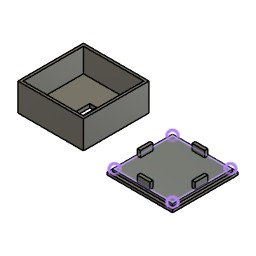
caja control servo_ (Autodesk Fusion 360 design; units mm, degrees)
Autodesk Fusion 360 part; units mm, degrees
sketch "Sketch1" plane through (0, 0, 0) normal (0, 1, 0) x (1, 0, 0)
  line L0 (-58.5421, 52.4156) -> (41.4579, 52.4156)
  line L1 (41.4579, 52.4156) -> (41.4579, -47.5844)
  line L2 (41.4579, -47.5844) -> (-58.5421, -47.5844)
  line L3 (-58.5421, -47.5844) -> (-58.5421, 52.4156)
  dimension "d1" = 100
  dimension "d2" = 100
  constraint horizontal L0
  constraint vertical L1
  constraint horizontal L2
  constraint vertical L3
  measures "d1" distance of L0.start L0.end
  measures "d2" distance of L0.start L2.end
extrude "Extrude1" add sketch "Sketch1" along normal blind 40 makes body 1
shell "Shell1" thickness 2 outward thickness 2 removed faces 1 at (-25.2087, 40, -19.0822) on bodies 1
sketch "Sketch2" plane through (0, 2, 0) normal (0, 1, 0) x (-1, 0, 0)
  line L0 (56.5421, 45.5844) -> (-39.4579, 45.5844)
  line L1 (-39.4579, 45.5844) -> (-39.4579, -50.4156)
  line L2 (-39.4579, -50.4156) -> (56.5421, -50.4156)
  line L3 (56.5421, -50.4156) -> (56.5421, 45.5844)
  line L4 (0.5421, 9.5844) -> (0.5421, -14.4156)
  line L5 (8.5421, 9.5844) -> (0.5421, 9.5844)
  line L6 (8.5421, -14.4156) -> (0.5421, -14.4156)
  line L7 (8.5421, 9.5844) -> (8.5421, -14.4156)
extrude "Extrude2" cut sketch "Sketch2" against normal blind 20 contours L4 L5 L6 L7 bodies 1
extrude "Extrude3" add 1 faces at (-43.2087, -2, -6.4156) along direction (0, -1, 0) blind 2 on bodies 1 bodies 1
sketch "Sketch4" plane through (0, 0, 0) normal (0, 1, 0) x (1, 0, 0)
  line L0 (80, 50) -> (180, 50)
  line L1 (180, 50) -> (180, -50)
  line L2 (180, -50) -> (80, -50)
  line L3 (80, -50) -> (80, 50)
  dimension "d13" = 100
  dimension "d14" = 100
  constraint horizontal L0
  constraint vertical L1
  constraint horizontal L2
  constraint vertical L3
  measures "d13" distance of L0.start L0.end
  measures "d14" distance of L0.start L2.end
extrude "Extrude4" add sketch "Sketch4" along normal blind 2 separate body makes body 2
sketch "Sketch5" plane through (0, 2, 0) normal (0, 1, 0) x (-1, 0, 0)
  line L0 (-80, 50) -> (-180, 50)
  line L1 (-180, 50) -> (-180, -50)
  line L2 (-180, -50) -> (-80, -50)
  line L3 (-80, -50) -> (-80, 50)
  line L4 (-84, 46) -> (-176, 46)
  line L5 (-176, 46) -> (-176, -46)
  line L6 (-176, -46) -> (-84, -46)
  line L7 (-84, -46) -> (-84, 46)
  dimension "d17" = -4
extrude "Extrude5" add sketch "Sketch5" along normal blind 4 contours L4 L5 L6 L7 bodies 2
extrude "Extrude6" add 1 faces at (113.3333, 0, -16.6667) along direction (0, -1, 0) blind 2 on bodies 2 bodies 2
copy_body "Body->Comp1" bodies 2 removing the originals makes body 3 in component "Component"
copy_body "Body->Comp2" bodies 1 removing the originals makes body 4 in component "Component'"
sketch "Sketch6" plane through (0, 6, 0) normal (0, 1, 0) x (-1, 0, 0)
  line L0 (-84, -46) -> (-84, 46)
  line L1 (-84, 46) -> (-176, 46)
  line L2 (-176, 46) -> (-176, -46)
  line L3 (-176, -46) -> (-84, -46)
sketch "Sketch7" plane through (0, 6, 0) normal (0, 1, 0) x (-1, 0, 0)
  line L0 (-84, -46) -> (-84, 46)
  line L1 (-84, 0) -> (-84, -10)
  line L2 (-84, -10) -> (-89, -10)
  line L3 (-89, -10) -> (-89, 10)
  line L4 (-89, 10) -> (-84, 10)
  line L5 (-84, 10) -> (-84, -10)
  dimension "d22" = 10
  dimension "d23" = 5
  dimension "d24" = 20
  constraint midpoint L0 L1.start
  constraint parallel L0 L1
  constraint horizontal L2
  constraint vertical L3
  constraint horizontal L4
  constraint vertical L5
  measures "d22" distance of L1.start L1.end
  measures "d23" distance of L1.end L2.end
  measures "d24" distance of L1.end L4.end
extrude "Extrude7" add sketch "Sketch7" along normal blind 10 separate body makes body 5
sketch "Sketch8" plane through (0, 6, 0) normal (0, 1, 0) x (-1, 0, 0)
  line L0 (-176, -46) -> (-84, -46)
  line L1 (-84, 46) -> (-176, 46)
sketch "Sketch9" plane through (0, 6, 0) normal (0, 1, 0) x (-1, 0, 0)
  line L0 (-84, -46) -> (-84, 46)
  line L1 (-176, 46) -> (-176, -46)
sketch "Sketch10" plane through (0, 6, 0) normal (0, 1, 0) x (-1, 0, 0)
  line L0 (-130, -46) -> (-120, -46)
  line L1 (-120, -46) -> (-140, -46)
  line L2 (-140, -46) -> (-140, -41)
  line L3 (-140, -41) -> (-120, -41)
  line L4 (-120, -41) -> (-120, -46)
  line L5 (-176, 0) -> (-176, -10)
  line L6 (-176, -10) -> (-171, -10)
  line L7 (-171, -10) -> (-171, 10)
  line L8 (-171, 10) -> (-176, 10)
  line L9 (-176, 10) -> (-176, -10)
  line L10 (-130, 46) -> (-140, 46)
  line L11 (-140, 46) -> (-120, 46)
  line L12 (-120, 46) -> (-120, 41)
  line L13 (-120, 41) -> (-140, 41)
  line L14 (-140, 41) -> (-140, 46)
  point P0 (-130, -46)
  point P1 (-176, 0)
  point P2 (-130, 46)
  dimension "d27" = 10
  dimension "d28" = 20
  dimension "d29" = 5
  dimension "d30" = 10
  dimension "d31" = 5
  dimension "d32" = 20
  dimension "d33" = 10
  dimension "d34" = 20
  dimension "d35" = 5
  constraint coincident P0 L0.start
  constraint horizontal L1
  constraint vertical L2
  constraint horizontal L3
  constraint vertical L4
  constraint coincident P1 L5.start
  constraint perpendicular L1 L5
  constraint horizontal L6
  constraint vertical L7
  constraint horizontal L8
  constraint vertical L9
  constraint coincident P2 L10.start
  constraint horizontal L11
  constraint vertical L12
  constraint horizontal L13
  constraint vertical L14
  measures "d27" distance of P0 L0.end
  measures "d28" distance of L0.end L1.end
  measures "d29" distance of L0.end L3.end
  measures "d30" distance of P1 L5.end
  measures "d31" distance of L5.end L6.end
  measures "d32" distance of L5.end L8.end
  measures "d33" distance of P2 L10.end
  measures "d34" distance of L10.end L11.end
  measures "d35" distance of L10.end L13.end
extrude "Extrude8" add sketch "Sketch10" along normal blind 10 separate body makes body 6 at (126.6667, 9.3333, -46) makes body 7 at (176, 9.3333, 3.3333) makes body 8 at (133.3333, 9.3333, 46)
extrude "Extrude1'" add 1 faces at (80, 0.6667, 16.6667) along direction (-1, 0, 0) blind 2 on bodies 3 bodies 3 in component "Component"
extrude "Extrude2'" add 1 faces at (180, -0.6667, 16.6667) along direction (1, 0, 0) blind 2 on bodies 3 bodies 3 in component "Component"
extrude "Extrude3'" add 1 faces at (112.6667, 0.6667, 50) along direction (0, 0, 1) blind 2 on bodies 3 bodies 3 in component "Component"
extrude "Extrude4'" add 1 faces at (147.3333, -0.6667, -50) along direction (0, 0, -1) blind 2 on bodies 3 bodies 3 in component "Component"
extrude "Extrude5'" add 1 faces at (84, 3.3333, -15.3333) along direction (-1, 0, 0) blind 1.5 on bodies 3 bodies 3 in component "Component"
extrude "Extrude6'" add 1 faces at (113.6667, 4.6667, -46) along direction (0, 0, -1) blind 1.5 on bodies 3 bodies 3 in component "Component"
extrude "Extrude7'" add 1 faces at (176, 3.3333, 14.8333) along direction (1, 0, 0) blind 1.5 on bodies 3 bodies 3 in component "Component"
extrude "Extrude8'" add 1 faces at (145.8333, 4.6667, 46) along direction (0, 0, 1) blind 1.5 on bodies 3 bodies 3 in component "Component"
combine "Combine1" operation add target body 3 tool bodies 6 7 8 in component "Component"
extrude "Extrude1''" cut 1 faces at (-8.5421, 0, 1.5844) along direction (-1, 0, 0) blind 2 on bodies 4 bodies 4 in component "Component'"
extrude "Extrude2''" cut 1 faces at (-7.2087, 0, 9.5844) along direction (0, 0, 1) blind 1.5 on bodies 4 bodies 4 in component "Component'"
extrude "Extrude3''" cut 1 faces at (-0.5421, 0, 2.5844) along direction (1, 0, 0) blind 1 on bodies 4 bodies 4 in component "Component'"
component "Component" placed x (1, 0, 0) y (0, 1, 0) z (0, 0, 1) at (0, 0, 0)
component "Component'" placed x (1, 0, 0) y (0, 1, 0) z (0, 0, 1) at (-17.0945, 2.3227, -11.6882)
